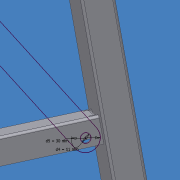
# Autodesk Inventor part: 90-08-0850
Saved by Autodesk Inventor 2015 (Build 190159000, 159)
## iProperties
Created: 2007-08-02
Part Number: 90-08-0850
Material: Steel, Mild
Document SubType Name: Modeling
Designer: kurt
Manufacturer: Standard
Standards Organization: Custom
Density: 7.86 g/cm^3
Appearance: Steel
Behandeling: Behandeling
Besteld: S
Materiaal: st37
Totaal: 0
Author: kurt
Autodesk Inventor part; units mm, degrees
ref_plane "YZ Plane" through (0, 0, 0) normal (1, 0, 0) x (0, 1, 0)
ref_plane "XZ Plane" through (0, 0, 0) normal (0, 1, 0) x (-1, 0, 0)
ref_plane "XY Plane" through (0, 0, 0) normal (0, 0, 1) x (1, 0, 0)
sketch "Sketch1" plane through (0, 0, 0) normal (0, 0, 1) x (1, 0, 0)
  circle A0 centre (192, 3.5) radius 5.5 projected
  circle A1 centre (-192, 633) radius 5.5 projected
  circle A2 centre (-192, 633) radius 5.5
  arc A3 (-179.1945, 640.8115) -> (-204.8055, 625.1885) centre (-192, 633) ccw
  circle A4 centre (192, 3.5) radius 5.5
  arc A5 (179.1945, -4.3115) -> (204.8055, 11.3115) centre (192, 3.5) ccw
  line L0 (-179.1945, 640.8115) -> (204.8055, 11.3115)
  line L1 (179.1945, -4.3115) -> (-204.8055, 625.1885)
  point P0 (0, 0)
  dimension "d2" = 30
  dimension "d3" = 11
  dimension "d4" = 11
  dimension "d5" = 30
  constraints: 4 centre point, 4 coincident, 4 end point, 4 point on circle, 4 tangent
  measures "d2" diameter of A5
  measures "d3" diameter of A4
  measures "d4" diameter of A2
  measures "d5" diameter of A3
extrude "Extrusion2" add sketch "Sketch1" along normal blind 6
body "Solid1"
